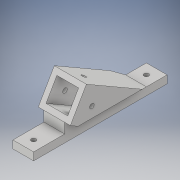
# Autodesk Inventor part: 30DegreeAttachementV03
Saved by Autodesk Inventor 2019.3 (Build 233278000, 278)
## iProperties
Created: 2019-02-16
Part Number: 30DegreeAttachementV03
Material: Generic
Document SubType Name: Modeling
Designer: steele
Density: 1 g/cm^3
Appearance: Default
Author: steele
Autodesk Inventor part; units mm, degrees
ref_plane "YZ Plane" through (0, 0, 0) normal (1, 0, 0) x (0, 1, 0)
ref_plane "XZ Plane" through (0, 0, 0) normal (0, 1, 0) x (-1, 0, 0)
ref_plane "XY Plane" through (0, 0, 0) normal (0, 0, 1) x (1, 0, 0)
sketch "Sketch1" plane through (0, 0, 0) normal (1, 0, 0) x (0, 1, 0)
  line L0 (0, 0) -> (12.4509, 21.5656)
  line L1 (12.4509, 21.5656) -> (46.5463, 1.8806)
  line L2 (0, -101.8491) -> (0, 42.1347) projected
  line L3 (46.5463, 1.8806) -> (0, -78.74)
  line L4 (0, 0) -> (0, -78.74)
  line L5 (19.05, 17.7556) -> (0, -15.24) construction
  dimension "d0" = 39.37
  dimension "d1" = 30
  dimension "d5" = 7.62
  dimension "d6" = 38.1
  constraints: 10 end point, 3 point on line, 2 parallel, 1 collinear, 1 perpendicular
  measures "d0" distance of L0.end L1.end
  measures "d1" angle of L0 L2
  measures "d5" distance between parallel lines of L5 L0
  measures "d6" distance from line of L5.end L1
extrude "Extrusion1" add sketch "Sketch1" along normal mid plane 39.37
sketch "Sketch2" plane through (-19.685, 12.4509, 21.5656) normal (0, 0.5, 0.866) x (1, 0, 0)
  line L0 (0, 0) -> (39.37, 0) construction
  line L1 (39.37, 0) -> (39.37, 39.37) construction
  line L2 (0, 0) -> (39.37, 39.37) construction
  line L3 (39.37, 39.37) -> (0, 39.37) construction
  line L4 (0, 39.37) -> (39.37, 0) construction
  line L5 (6.35, 6.35) -> (33.02, 6.35)
  line L6 (33.02, 6.35) -> (33.02, 33.02)
  line L7 (33.02, 33.02) -> (6.35, 33.02)
  line L8 (6.35, 33.02) -> (6.35, 6.35)
  line L9 (6.35, 6.35) -> (33.02, 33.02) construction
  line L10 (33.02, 6.35) -> (6.35, 33.02) construction
  point P0 (19.685, 0)
  point P1 (19.685, 19.685)
  dimension "d7" = 26.67
  constraints: 16 end point, 3 midpoint, 2 parallel, 2 perpendicular, 1 horizontal
  measures "d7" distance of L7.end L5.start
extrude "Extrusion2" cut sketch "Sketch2" against normal blind 38.1
sketch "Sketch3" plane through (0, 0, 0) normal (1, 0, 0) x (0, 1, 0)
  line L0 (12.4509, 21.5656) -> (0, 0) projected
  line L1 (0, 0) -> (0, -78.74) projected
  line L2 (0, -78.74) -> (46.5463, 1.8806) projected
  line L3 (21.997, -27.94) -> (0, -15.24) projected
  line L4 (17.9501, 18.3906) -> (0, -12.7) projected
  line L5 (0, 0) -> (0, -78.74)
  line L6 (12.4509, 21.5656) -> (-1.0999, 21.5656) construction
  line L7 (0, 0) -> (12.4509, 21.5656) projected
  line L8 (0, 0) -> (0, 59.6656)
  line L9 (46.5463, 1.8806) -> (0, -78.74) projected
  line L10 (0, -78.74) -> (0, -104.14)
  line L11 (0, -137.4091) -> (0, 77.6947) projected
  line L12 (0, 59.6656) -> (-9.525, 59.6656)
  line L13 (-9.525, 59.6656) -> (-9.525, -104.14)
  line L14 (-9.525, -104.14) -> (0, -104.14)
  point P0 (1.0999, -13.335)
  point P1 (0, -15.24)
  point P2 (0, -12.7)
  dimension "d10" = 38.1
  dimension "d11" = 25.4
  dimension "d12" = 9.525
  dimension "supportBaseLength" = 163.8056
  constraints: 14 end point, 5 vertical, 2 horizontal, 2 perpendicular, 3 other
  measures "d10" distance from line of L8.end L6
  measures "d11" distance of L1.end L10.end
  measures "d12" distance of L8.end L12.end
  measures "supportBaseLength" distance between parallel lines of L14 L12
extrude "Extrusion3" add sketch "Sketch3" along normal mid plane 25.4
sketch "Sketch5" plane through (0, 0, 0) normal (1, 0, 0) x (0, 1, 0)
  line L0 (0, 0) -> (12.4509, 21.5656) projected
  line L1 (0, 59.6656) -> (0, 0) projected
  line L2 (12.4509, 21.5656) -> (46.5463, 1.8806) projected
  line L3 (12.4509, 21.5656) -> (0, 21.5656)
  line L4 (0, 0) -> (12.4509, 21.5656)
  constraints: 4 end point, 1 horizontal, 1 point on line
extrude "Extrusion5" add sketch "Sketch5" along normal mid plane 25.4
sketch "Sketch4" plane through (0, 0, 0) normal (0, 0, 1) x (1, 0, 0)
  line L0 (19.685, 46.5463) -> (-19.685, 46.5463) projected
  line L1 (19.685, 0) -> (19.685, 46.5463) projected
  line L2 (19.685, 0) -> (12.7, 0) projected
  line L3 (12.7, 0) -> (-12.7, 0) projected
  line L4 (-12.7, 0) -> (-19.685, 0) projected
  line L5 (-19.685, 46.5463) -> (-19.685, 0) projected
  line L6 (-12.7, 0) -> (-12.7, -9.525) projected
  line L7 (12.7, -9.525) -> (-12.7, -9.525) projected
  line L8 (12.7, -9.525) -> (12.7, 0) projected
  line L9 (-12.7, 0) -> (-19.685, 6.985)
  line L10 (-19.685, 46.5463) -> (-19.685, 0) projected
  line L11 (-19.685, 6.985) -> (-19.685, 0)
  line L12 (0, 0) -> (0, 46.5463) construction
  line L13 (12.7, 0) -> (19.685, 0)
  line L14 (12.7, 0) -> (19.685, 6.985)
  line L15 (19.685, 6.985) -> (19.685, 0)
  dimension "d15" = 45
  constraints: 12 end point, 1 collinear, 1 midpoint, 1 point on line, 1 symmetric about line
  measures "d15" angle of L9 L4
extrude "Extrusion4" cut sketch "Sketch4" against normal up to surface (163.8056 mm away) from surface at 59.6656 contours L1 L2 L14 | L9 L4 L5
sketch "Sketch6" plane through (-12.7, 0, 59.6656) normal (0, 1, 0) x (1, 0, 0)
  line L0 (25.4, 163.8056) -> (0, 163.8056) construction
  line L1 (12.7, 163.8056) -> (12.7, 0) construction
  line L2 (25.4, 0) -> (0, 0) construction
  point P0 (12.7, 59.6656)
  point P1 (12.7, 151.1056)
  point P2 (12.7, 12.7)
  dimension "d21" = 12.7
  dimension "d22" = 12.7
  constraints: 2 end point, 2 midpoint, 2 point on line
  measures "d21" distance from line of point (12.7, 12.7) L2
  measures "d22" distance from line of point (12.7, 151.106) L0
hole "Hole1" at (0, 0, -91.44) at (0, 0, 46.9656) direction (0, -1, 0) diameter 5.6134 end through all clearance for "Flat Head Machine Screw (82)" size "#10" standard "Ansi Unified Screw Threads"
sketch "Sketch9" plane through (0, 0, 0) normal (1, 0, 0) x (0, 1, 0)
  line L0 (0.635, -11.6001) -> (0.635, -15.6066) projected
  line L1 (0.635, -15.6066) -> (21.997, -27.94) projected
  line L2 (41.047, 5.0556) -> (21.997, -27.94) projected
  line L3 (17.9501, 18.3906) -> (41.047, 5.0556) projected
  line L4 (17.9501, 18.3906) -> (0.635, -11.6001) projected
  line L5 (29.4986, 11.7231) -> (10.4486, -21.2725) construction
  line L6 (0.635, -15.6066) -> (21.997, -27.94) construction
  circle A0 centre (19.9736, -4.7747) radius 2.8067
  point P0 (0, 0)
  dimension "d30" = 5.6134
  constraints: 2 end point, 2 midpoint, 1 centre point, 1 perpendicular, 1 point on line
  measures "d30" diameter of A0
extrude "Extrusion6" cut sketch "Sketch9" along normal through all both and the other way through all contours A0
sketch "Sketch10" plane through (-19.685, 46.5463, 1.8806) normal (0, 0.866, -0.5) x (1, 0, 0)
  line L0 (6.35, 0) -> (33.02, 0) construction
  line L1 (19.685, 0) -> (19.685, 77.7875) construction
  point P0 (19.685, 24.9018)
  point P1 (19.685, 19.05)
  dimension "d33" = 19.05
  constraints: 2 end point, 1 midpoint, 1 point on line, 1 vertical
  measures "d33" distance from line of point (19.685, 19.05) L0
hole "Hole2" at (0, 37.0213, -14.6172) direction (0, -0.866, 0.5) diameter 5.6134 depth 6.35 clearance for "Flat Head Machine Screw (82)" size "#10" standard "Ansi Unified Screw Threads"
equation "\"d0\" = widthToSupportExtrusion"
equation "\"d1\" = attachementAngle"
equation "\"d6\" = insertDepth"
equation "\"d2\" = widthToSupportExtrusion"
equation "\"d7\" = insertForExtrusion"
equation "\"d8\" = insertDepth"
equation "\"d10\" = lenghtUnderBrace"
equation "\"d11\" = backLength"
equation "\"d12\" = supportBaseDepth"
equation "\"d13\" = supportBaseWidth"
equation "\"d19\" = supportBaseWidth"
equation "\"d21\" = supportHoleDistanceFromEnd"
equation "\"d22\" = supportHoleDistanceFromEnd"
equation "\"attachementAngle\" = 30deg"
equation "\"extrusionSize\" = 25.4"
equation "\"wallThickness\" = 6.35"
equation "\"slipClearance\" = 0.635"
equation "\"insertForExtrusion\" = extrusionSize + 2 * slipClearance"
equation "\"widthToSupportExtrusion\" = insertForExtrusion + 2 * wallThickness"
equation "\"insertDepth\" = 38.1"
equation "\"supportBaseWidth\" = 25.4"
equation "\"supportBaseDepth\" = 9.525"
equation "\"supportHoleDistanceFromEnd\" = 12.7"
equation "\"lenghtUnderBrace\" = 38.1"
equation "\"backLength\" = 25.4"
body "Solid1"
